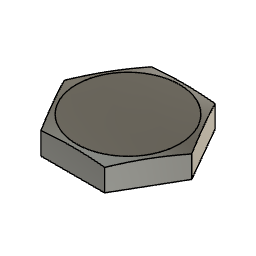
Leading Wheel Holder (Autodesk Fusion 360 design; units mm, degrees)
Autodesk Fusion 360 part; units mm, degrees
sketch "Sketch1" plane through (0, 0, 0) normal (0, 0, 1) x (1, 0, 0) in component "Component"
  circle A0 centre (0, 0) radius 1.05
  line L0 (-1.299, 2.25) -> (-2.5981, 0)
  line L1 (-2.5981, 0) -> (-1.299, -2.25)
  line L2 (-1.299, -2.25) -> (1.299, -2.25)
  line L3 (1.299, -2.25) -> (2.5981, 0)
  line L4 (2.5981, 0) -> (1.299, 2.25)
  line L5 (1.299, 2.25) -> (-1.299, 2.25)
  dimension "d1" = 2.1
  dimension "d3" = 2.25
  constraint coincident A0.centre origin
  measures "d1" diameter of A0
  measures "d3" distance of A0.centre L5
extrude "Extrude1" add sketch "Sketch1" along normal blind 1 contours A0 | L0 L1 L2 L3 L4 L5 in component "Component"
extrude "Extrude2" cut sketch "Sketch1" along normal blind 0.3 contours A0 in component "Component"
sketch "Sketch2" plane through (0, 0, 0) normal (1, 0, 0) x (0, 1, 0) in component "Component"
  line L0 (2.1, 1) -> (3.0799, 0.8006)
  line L1 (2.1, 1) -> (3.1, 1) construction
  line L2 (3.0799, 0.8006) -> (3.1, 1)
  line L3 (2.1, 1) -> (3.1, 1)
  dimension "d8" = 1
  dimension "d9" = 11.5
  constraint horizontal L1
  constraint parallel L1 L3
  measures "d8" distance of L0.start L0.end
  measures "d9" angle of L0 L1
revolve "Revolve1" cut sketch "Sketch2" angle 360 about axis through (0, 0, 1.75) along (0, 0, 1) in component "Component"
component "Component" placed x (1, 0, 0) y (0, 1, 0) z (0, 0, 1) at (0, 0, 0)
